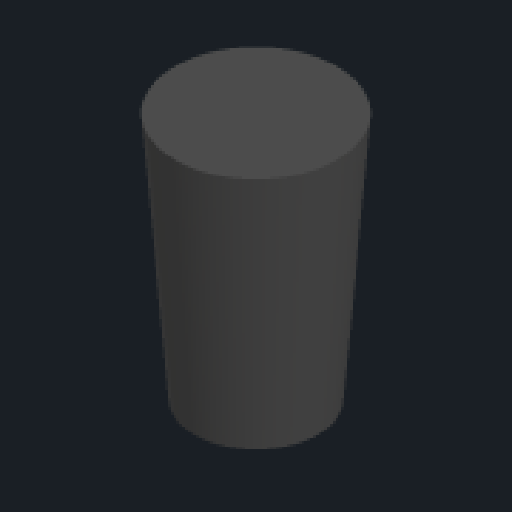
# Autodesk Inventor part: SC-1-01-Test Tube Cap
Saved by Autodesk Inventor 2023.1 (Build 271208000, 208)
## iProperties
Created: 2023-02-20
Part Number: SC-1-01-Test Tube Cap
Material: Rubber
Document SubType Name: Modeling
Designer: annah
Density: 0.93 g/cm^3
Appearance: Rubber - Black
Author: annah
Autodesk Inventor part; units mm, degrees
ref_plane "YZ Plane" through (0, 0, 0) normal (1, 0, 0) x (0, 1, 0)
ref_plane "XZ Plane" through (0, 0, 0) normal (0, 1, 0) x (-1, 0, 0)
sketch "Sketch1" plane through (0, 0, 0) normal (0, 1, 0) x (-1, 0, 0)
  circle A0 centre (0, 0) radius 8.5
  dimension "d0" = 17
  constraints: 1 centre point, 1 coincident
  measures "d0" diameter of A0
ref_plane "Work Plane1" through (0, 0, 0) normal (0, -1, 0) x (1, 0, 0)
ref_plane "Work Plane2" through (0, -25.94, 0) normal (0, -1, 0) x (1, 0, 0)
sketch "Sketch4" plane through (0, -25.94, 0) normal (0, -1, 0) x (1, 0, 0)
  circle A0 centre (0, 0) radius 6.5
  dimension "d5" = 13
  constraints: 1 centre point, 1 coincident
  measures "d5" diameter of A0
loft "Loft1" add profiles "Sketch1", "Sketch4"
body "Solid2"
